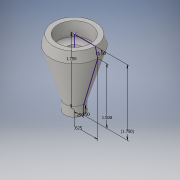
# Autodesk Inventor part: Sun_Stack
Saved by Autodesk Inventor 2016 (Build 200138000, 138)
## iProperties
Created: 2018-01-09
Part Number: Sun_Stack
Material: Generic
Document SubType Name: Modeling
Designer: sun01147
Density: 1 g/cm^3
Appearance: Default
Mass: 12.5845 g
Surface Area: 54.7818 cm^2
Volume: 12.5845 cm^3
Author: sun01147
Autodesk Inventor part; units mm, degrees
ref_plane "XZ Plane" through (0, 0, 0) normal (0, 1, 0) x (-1, 0, 0)
ref_plane "XY Plane" through (0, 0, 0) normal (0, 0, 1) x (1, 0, 0)
sketch "Sketch1" plane through (0, 0, 0) normal (0, 0, 1) x (1, 0, 0)
  line L0 (0, 0) -> (6.35, 0)
  line L1 (6.35, 0) -> (6.35, 6.35)
  line L2 (0, 0) -> (0, 44.45)
  line L3 (0, 44.45) -> (14.1735, 44.45)
  line L4 (6.35, 6.35) -> (15.875, 38.1)
  line L5 (15.875, 38.1) -> (14.1735, 44.45)
  dimension "d0" = 6.35
  dimension "d1" = 6.35
  dimension "d2" = 44.45
  dimension "d4" = 38.1
  dimension "d5" = 44.45
  dimension "d6" = 15.875
  dimension "d7" = 75
  constraints: 12 end point, 2 horizontal, 2 vertical
  measures "d0" distance of L0.start L0.end
  measures "d1" distance of L0.end L1.end
  measures "d2" distance of L0.start L2.end
  measures "d4" vertical distance of L0.end L4.end
  measures "d5" vertical distance of L0.end L3.end
  measures "d6" distance from line of L2 L4.end
  measures "d7" angle of L3 L5
revolve "Revolution1" add sketch "Sketch1" angle 360 about axis through (0, 0, 0) along (0, 1, 0)
sketch "Sketch2" plane through (0, 44.45, 0) normal (0, 1, 0) x (1, 0, 0)
  point P0 (0, 0)
  point P1 (0, 0)
  constraints: 1 coincident
hole "Hole1" at (0, 44.45, 0) direction (0, -1, 0) diameter 9.525 depth 38.1 tip angle 118 counterbore diameter 22.225 counterbore depth 9.525
body "Solid1"
